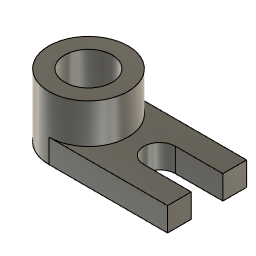
ch3Example-video v1 (Autodesk Fusion 360 design; units mm, degrees)
Autodesk Fusion 360 part; units mm, degrees
sketch "Sketch1" plane through (0, 0, 0) normal (0, 0, 1) x (1, 0, 0) in component "CSGexample"
  line L0 (0, 50) -> (75, 50)
  line L1 (75, 50) -> (75, 0)
  line L2 (75, 0) -> (0, 0)
  line L3 (0, 0) -> (0, 50)
  dimension "d1" = 75
  dimension "d2" = 50
  constraint horizontal L0
  constraint vertical L1
  constraint horizontal L2
  constraint vertical L3
  constraint coincident L2.end L3.start
  measures "d1" distance of L0.start L0.end
  measures "d2" distance of L0.start L2.end
extrude "Extrude1" add sketch "Sketch1" along normal blind 15 in component "CSGexample"
sketch "Sketch2" plane through (0, 0, 0) normal (0, 0, -1) x (1, 0, 0) in component "CSGexample"
  line L0 (75, 0) -> (0, 0)
  line L1 (0, 0) -> (0, -50)
  line L2 (0, -50) -> (75, -50)
  line L3 (75, -50) -> (75, 0)
  circle A0 centre (0, -25) radius 25
  constraint coincident L0.end A0
  constraint tangent L0 A0
  constraint coincident L1.end A0
extrude "Extrude2" add sketch "Sketch2" against normal blind 40 contours L1 A0 | L1 A0 in component "CSGexample"
sketch "Sketch3" plane through (0, 0, 40) normal (0, 0, 1) x (-1, 0, 0) in component "CSGexample"
  circle A0 centre (0, -25) radius 25
  circle A1 centre (0, -25) radius 15
  dimension "d7" = 30
  constraint concentric A0 A1
  measures "d7" diameter of A1
extrude "Extrude3" cut sketch "Sketch3" against normal through all contours A1 in component "CSGexample"
hole "Hole1" at (45, 25, 15) direction (0, 0, -1) diameter 20 end through all in component "CSGexample"
sketch "Sketch4" plane through (75, 0, 0) normal (1, 0, 0) x (0, 1, 0) in component "CSGexample"
  line L0 (0, 0) -> (50, 0)
  line L1 (50, 0) -> (50, 15)
  line L2 (50, 15) -> (0, 15)
  line L3 (0, 15) -> (0, 0)
  line L4 (15, 15) -> (35, 15)
  line L5 (35, 15) -> (35, 0)
  line L6 (35, 0) -> (15, 0)
  line L7 (15, 0) -> (15, 15)
  dimension "d15" = 20
  constraint horizontal L4
  constraint vertical L5
  constraint horizontal L6
  constraint vertical L7
  constraint coincident L0 L5.end
  constraint coincident L2 L4.start
  constraint midpoint L0 L6
  measures "d15" distance of L5.end L6.end
extrude "Extrude4" cut sketch "Sketch4" along normal up to surface contours L0 L2 L4 L5 L6 L7 end surface at (45.9957, 15.0497, 10) in component "CSGexample"
component "CSGexample" placed x (1, 0, 0) y (0, 1, 0) z (0, 0, 1) at (0, 0, 0)
